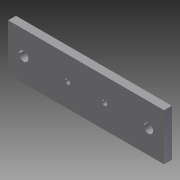
# Autodesk Inventor part: z axis mount
Saved by Autodesk Inventor 2011 (Build 150239000, 239)
## iProperties
Created: 2014-03-28
Part Number: z axis mount
Document SubType Name: Modeling
Designer: Devon
Density: 1 g/cm^3
Author: Devon
Autodesk Inventor part; units mm, degrees
ref_plane "YZ Plane" through (0, 0, 0) normal (1, 0, 0) x (0, 1, 0)
ref_plane "XZ Plane" through (0, 0, 0) normal (0, 1, 0) x (-1, 0, 0)
ref_plane "XY Plane" through (0, 0, 0) normal (0, 0, 1) x (1, 0, 0)
sketch "Sketch1" plane through (0, 0, 0) normal (0, 0, 1) x (1, 0, 0)
  line L0 (-76.9591, 41.6961) -> (50.0409, 41.6961)
  line L1 (50.0409, 41.6961) -> (50.0409, 3.5961)
  line L2 (50.0409, 3.5961) -> (-76.9591, 3.5961)
  line L3 (-76.9591, 3.5961) -> (-76.9591, 41.6961)
  circle A0 centre (-28.4591, 22.6461) radius 2.0193
  circle A1 centre (1.5409, 22.6461) radius 2.0193
  circle A2 centre (-64.2591, 22.6461) radius 3.81
  circle A3 centre (37.3409, 22.6461) radius 3.81
  point P0 (0, 0)
  dimension "d0" = 127
  dimension "d1" = 38.1
  dimension "d4" = 4.0386
  dimension "d5" = 4.0386
  dimension "d8" = 7.62
  dimension "d9" = 7.62
  constraints: 8 end point, 4 centre point, 2 parallel, 1 horizontal, 1 perpendicular
  measures "d0" distance of L1.end L2.end
  measures "d1" distance of L0.end L1.end
  measures "d4" diameter of A0
  measures "d5" diameter of A1
  measures "d8" diameter of A2
  measures "d9" diameter of A3
extrude "Extrusion1" add sketch "Sketch1" along normal blind 6.35
body "Solid1"
